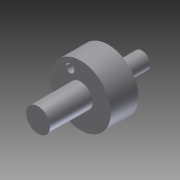
# Autodesk Inventor part: Post
Saved by Autodesk Inventor 2011 SP2 (Build 150309200, 309)
## iProperties
Created: 2013-02-08
Part Number: Post
Document SubType Name: Modeling
Designer: sungwook
Density: 1 g/cm^3
Author: sungwook
Autodesk Inventor part; units mm, degrees
ref_plane "YZ Plane" through (0, 0, 0) normal (1, 0, 0) x (0, 1, 0)
ref_plane "XZ Plane" through (0, 0, 0) normal (0, 1, 0) x (-1, 0, 0)
ref_plane "XY Plane" through (0, 0, 0) normal (0, 0, 1) x (1, 0, 0)
sketch "Sketch1" plane through (0, 0, 0) normal (0, 0, 1) x (1, 0, 0)
  circle A0 centre (0, 0) radius 2.159
  dimension "d0" = 4.318
  constraints: 1 centre point, 1 coincident
  measures "d0" diameter of A0
extrude "Extrusion1" add sketch "Sketch1" along normal blind 12.7
sketch "Sketch2" plane through (0, 0, 0) normal (0, 0, -1) x (-1, 0, 0)
  circle A0 centre (0, 0) radius 2.159 projected
  circle A1 centre (0, 0) radius 1.4986
  dimension "d3" = 2.9972
  constraints: 1 centre point, 1 coincident
  measures "d3" diameter of A1
extrude "Extrusion2" add sketch "Sketch2" along normal blind 6.096 contours A1
sketch "Sketch3" plane through (0, 0, 0) normal (0, 0, -1) x (-1, 0, 0)
  circle A0 centre (0, 0) radius 2.159 projected
  circle A1 centre (0, 0) radius 5.461
  dimension "d6" = 10.922
  constraints: 1 centre point, 1 coincident
  measures "d6" diameter of A1
extrude "Extrusion3" add sketch "Sketch3" against normal blind 5
sketch "Sketch4" plane through (0, 0, 5) normal (0, 0, 1) x (1, 0, 0)
  circle A0 centre (0, 0) radius 2.159 projected
  line L0 (-7.6454, 0) -> (7.6454, 0) projected
  point P0 (3.81, 0)
  point P1 (-1.905, 3.2996)
  point P2 (-1.905, -3.2996)
  dimension "d9" = 3.81
  dimension "d12" = 360
  constraints: 1 point on line, 4 other
  measures "d9" distance of A0.centre point (3.81, 0)
hole "Hole1" at (-1.905, 3.2996, 5) at (-1.905, -3.2996, 5) direction (0, 0, -1) diameter 1.524 end through all
body "Solid1"
